fadercap (Autodesk Fusion 360 design; units mm, degrees)
Autodesk Fusion 360 part; units mm, degrees
note: some values were not read from the file. Set by a fixed rule: which sketch regions a step uses.
sketch "Sketch1" plane through (0, 0, 0) normal (0, 1, 0) x (1, 0, 0)
  line L0 (0, 0) -> (13, 0)
  line L1 (13, 0) -> (13, -12)
  line L2 (13, -12) -> (0, -12)
  line L3 (0, -12) -> (0, 0)
  circle A0 centre (0, 0) radius 0.75
  circle A1 centre (0, -12) radius 0.75
  circle A2 centre (13, -12) radius 0.75
  circle A3 centre (13, 0) radius 0.75
  line L4 (13, 0) -> (21.5, 0)
  line L5 (0, 0) -> (-8.5, 0)
  line L6 (0, 0) -> (0, 2)
  line L7 (13, 0) -> (13, 2)
  line L8 (0, -12) -> (0, -14)
  line L9 (13, -12) -> (13, -14)
  line L10 (13, -12) -> (21.5, -12)
  line L11 (0, -12) -> (-8.5, -12)
  line L12 (-8.5, 2) -> (21.5, 2)
  line L13 (21.5, 2) -> (21.5, -14)
  line L14 (21.5, -14) -> (-8.5, -14)
  line L15 (-8.5, -14) -> (-8.5, 2)
  line L16 (-8.5, 2) -> (-10.5, 2)
  line L17 (-10.5, 2) -> (-10.5, -14)
  line L18 (-10.5, -14) -> (-8.5, -14)
  line L19 (-8.5, -14) -> (-8.5, 2)
  line L20 (21.5, 2) -> (23.5, 2)
  line L21 (23.5, 2) -> (23.5, -14)
  line L22 (23.5, -14) -> (21.5, -14)
  line L23 (21.5, -14) -> (21.5, 2)
  line L24 (23.5, -14) -> (23.5, -10.5)
  line L25 (23.5, -10.5) -> (-10.5, -10.5)
  line L26 (23.5, 2) -> (23.5, -1.5)
  line L27 (23.5, -1.5) -> (-10.5, -1.5)
  line L28 (6, 0) -> (6, -12)
  line L29 (0, -6) -> (13, -6)
  line L30 (13, -6) -> (13, 5)
  line L31 (13, 5) -> (13, -17)
  line L32 (13, 5) -> (-10.5, 5)
  line L33 (13, -17) -> (-10.5, -17)
  line L34 (6, 0) -> (6, -12)
  dimension "d1" = 12
  dimension "d2" = 13
  dimension "d3" = 1.5
  dimension "d4" = 1.5
  dimension "d5" = 1.5
  dimension "d6" = 1.5
  dimension "d7" = 8.5
  dimension "d8" = 8.5
  dimension "d9" = 2
  dimension "d10" = 2
  dimension "d11" = 2
  dimension "d12" = 2
  dimension "d13" = 2
  dimension "d14" = 2
  dimension "d15" = 3.5
  dimension "d16" = 3.5
  dimension "d25" = 11
  dimension "d26" = 22
  constraint horizontal L0
  constraint vertical L1
  constraint horizontal L2
  constraint vertical L3
  constraint coincident L0.start L3.end
  constraint coincident L2.end L3.start
  constraint coincident L1.end L2.start
  constraint coincident L0.end L1.start
  constraint perpendicular L1 L4
  constraint perpendicular L3 L5
  constraint perpendicular L5 L6
  constraint perpendicular L0 L7
  constraint perpendicular L2 L8
  constraint perpendicular L2 L9
  constraint perpendicular L9 L10
  constraint perpendicular L3 L11
  constraint horizontal L12
  constraint vertical L13
  constraint horizontal L14
  constraint vertical L15
  constraint horizontal L16
  constraint vertical L17
  constraint horizontal L18
  constraint vertical L19
  constraint horizontal L20
  constraint vertical L21
  constraint horizontal L22
  constraint vertical L23
  constraint perpendicular L22 L24
  constraint horizontal L25
  constraint coincident L17 L25.end
  constraint perpendicular L20 L26
  constraint coincident L17 L27.end
  constraint perpendicular L17 L27
  constraint coincident L0 L28.start
  constraint coincident L2 L28.end
  constraint perpendicular L2 L28
  constraint midpoint L3 L29.start
  constraint midpoint L1 L29.end
  constraint perpendicular L29 L30
  constraint perpendicular L14 L31
  constraint perpendicular L17 L32
  constraint perpendicular L17 L33
  measures "d1" distance of L0.start L2.end
  measures "d2" distance of L0.start L0.end
  measures "d3" diameter of A0
  measures "d4" diameter of A1
  measures "d5" diameter of A2
  measures "d6" diameter of A3
  measures "d7" distance of L0.end L4.end
  measures "d8" distance of L0.start L5.end
  measures "d9" distance of L0.start L6.end
  measures "d10" distance of L0.end L7.end
  measures "d11" distance of L2.end L8.end
  measures "d12" distance of L1.end L9.end
  measures "d13" distance of L12.start L16.end
  measures "d14" distance of L12.end L20.end
  measures "d15" distance of L21.end L24.end
  measures "d16" distance of L20.end L26.end
  measures "d25" distance of L29.end L30.end
  measures "d26" distance of L30.end L31.end
extrude "Extrude1" add sketch "Sketch1" against normal blind 3 contours L0 A0 L6 | L0 L3 A0 | L3 A0 L5 | A0 L5 L6 | L0 A3 L7 L30 L31 | L0 L1 A3 L30 L31 | L1 A3 L4 L30 L31 | A3 L4 L7 L30 L31 | L2 L3 A1 | L3 A1 L11 | L2 A1 L8 | A1 L8 L11 | L1 A2 L10 L31 | L1 L2 A2 L31 | L2 A2 L9 L31 | A2 L9 L10 L31 makes body 1 at (-0.7463, -1, 11.9253) makes body 2 at (13.7463, -1, 11.9253) makes body 3 at (0.7463, -2, 0.0747) makes body 4 at (13.7463, -2, 0.0747)
extrude "Extrude2" add sketch "Sketch1" against normal blind 2 separate body contours L15 L17 L19 L25 L27 | L13 L21 L23 L25 L27 makes body 5 at (-8.5, -0.6667, 7.5) makes body 6 at (22.1667, 0, 4.5)
extrude "Extrude3" add sketch "Sketch1" against normal blind 5 contours L15 L16 L17 L19 L27 | L15 L17 L18 L19 L25 | L13 L20 L21 L23 L26 L27 | L13 L21 L22 L23 L24 L25 bodies 5 6
extrude "Extrude4" add sketch "Sketch1" along normal blind 2 separate body makes body 7
sketch "Sketch2" plane through (0, 0, 0) normal (0, 1, 0) x (1, 0, 0)
  line L0 (13, 5) -> (0, 5)
  line L1 (0, 5) -> (0, -17)
  line L2 (0, -17) -> (13, -17)
  line L3 (13, -17) -> (13, 5)
  constraint horizontal L0
  constraint vertical L1
  constraint horizontal L2
  constraint vertical L3
ref_plane "WorkPlane1" through (6.5, 2, 6) normal (0, 1, 0) x (1, 0, 0)
sketch "Sketch3" plane through (6.5, 2, 6) normal (0, 1, 0) x (1, 0, 0)
  line L0 (-6.5, 11) -> (6.5, 11)
  line L1 (6.5, 11) -> (6.5, -11)
  line L2 (6.5, -11) -> (-6.5, -11)
  line L3 (-6.5, -11) -> (-6.5, 11)
  constraint horizontal L0
  constraint vertical L1
  constraint horizontal L2
  constraint vertical L3
extrude "Extrude5" add sketch "Sketch3" along normal blind 15 separate body makes body 8
chamfer "Chamfer1" distance 2 distance2 15 2 edges at (0, 17, 6) (13, 17, 6) measured on face at (4.3333, 17, 2.3333) measured on face at (4.3333, 17, 2.3333) on bodies 8
fillet "Fillet1" radius 2 2 edges at (11, 17, 6) (2, 17, 6) on bodies 8
move_body "Move1" bodies 8 to x (1, 0, 0) y (0, 1, 0) z (0, 0, 1) at (0, 2, 0)
sketch "Sketch4" plane through (0, 2, 0) normal (0, 1, 0) x (-1, 0, 0)
  line L0 (-23.5, -2) -> (10.5, -2)
  line L1 (10.5, -2) -> (10.5, 14)
  line L2 (10.5, 14) -> (-23.5, 14)
  line L3 (-23.5, 14) -> (-23.5, -2)
  line L4 (-6.5, 6) -> (-6.5, -5)
  line L5 (-6.5, -5) -> (-6.5, 17)
  circle A0 centre (-6.5, 6) radius 3
  dimension "d36" = 6
  constraint coincident L4.start A0.centre
  measures "d36" diameter of A0
extrude "Extrude6" add sketch "Sketch4" along normal blind 3 contours L4 L5 A0 | L4 L5 A0 bodies 8 7
